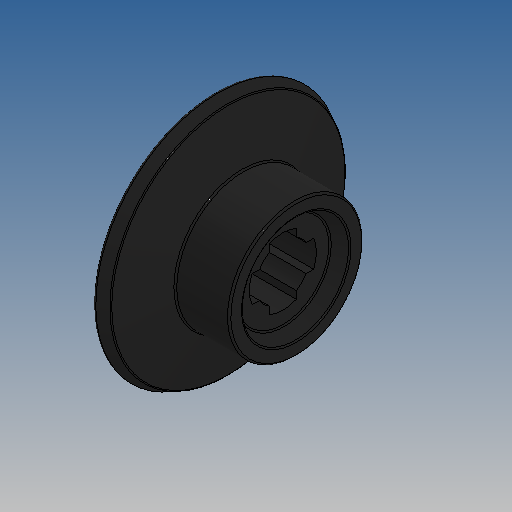
# Autodesk Inventor part: 50254-Black
Saved by Autodesk Inventor 2025 (Build 290162010, 162A)
## iProperties
Created: 2024-11-16
Part Number: 50254-Black
Material: ABS-Kunststoff
Document SubType Name: Modeling
Designer: hp.muther
Density: 1.06 g/cm^3
Appearance: Black
Author: hp.muther
Autodesk Inventor part; units mm, degrees
ref_plane "YZ Plane" through (0, 0, 0) normal (1, 0, 0) x (0, 1, 0)
ref_plane "XZ Plane" through (0, 0, 0) normal (0, 1, 0) x (-1, 0, 0)
ref_plane "XY Plane" through (0, 0, 0) normal (0, 0, 1) x (1, 0, 0)
sketch "Skizze1" plane through (0, 0, 0) normal (0, 1, 0) x (-1, 0, 0)
  line L0 (0, 0) -> (0, 7.2)
  line L1 (-0.1446, 7.2895) -> (-0.7422, 6.9916)
  line L2 (-0.7422, 6.9916) -> (-1.6, 4)
  line L3 (-1.6, 4) -> (-4.8, 4)
  line L4 (-4.8, 4) -> (-4.8, 0)
  line L5 (-4.8, 0) -> (0, 0)
  arc A0 (0, 7.2) -> (-0.1446, 7.2895) centre (-0.1, 7.2) ccw
  line L6 (-4.8, 3.1989) -> (-4, 2.8)
  line L7 (-4, 2.8) -> (-4, 0)
  line L8 (0, 2.4) -> (-0.7, 2.4)
  line L9 (-0.7979, 2.5201) -> (0, 6.4)
  arc A1 (-0.7979, 2.5201) -> (-0.7, 2.4) centre (-0.7, 2.5) ccw
  line L10 (0, 1.6) -> (-4, 1.6)
  dimension "d0" = 0.1
  dimension "d1" = 14.6
  dimension "d2" = 8
  dimension "d3" = 4.8
  dimension "d4" = 3.2
  dimension "d5" = 63.5
  dimension "d6" = 106
  dimension "d9" = 4.8
  dimension "d10" = 0.1
  dimension "d11" = 0.8
  dimension "d12" = 12.8
  dimension "d13" = 0.8
  dimension "d14" = 26.5
  dimension "d15" = 5.6
  dimension "d16" = 3.2
  constraints: 22 end point, 6 point on line, 4 point on circle, 4 tangent, 3 perpendicular, 2 centre point, 2 vertical, 1 horizontal, 1 parallel
  measures "d0" radius of A0
  measures "d2" diameter of L3 L5
  measures "d3" distance of L4.end L0.start
  measures "d4" distance of L2.end L3.end
  measures "d5" angle of L0 L1
  measures "d6" angle of L3 L2
  measures "d9" diameter of L8 L5
  measures "d10" radius of A1
  measures "d12" diameter of L9.end L5
  measures "d13" distance between parallel lines of L4 L7
  measures "d14" angle of L5 L6
  measures "d15" diameter of L6.end L5
  measures "d16" diameter of L10 L5
revolve "Umdrehung1" add sketch "Skizze1" angle 360 about axis through (4.8, 0, 0) along (-1, 0, 0) contours L10 L7 L6 L4 L3 L2 L1 A0 L0 L9 A1 L8
fillet "Rundung1" radius 0.1 7 edges at (4.8, 0, -4) (1.6, 0, -4) (0.7422, 0, -6.9916) (4.8, 0, -3.1989) (4, 0, -2.8) (0, 0, -2.4) (0, 0, -6.4)
sketch "Skizze2" plane through (0, 0, 0) normal (-1, 0, 0) x (0, 0, 1)
  circle A0 centre (0, 0) radius 2.3 projected
  line L0 (0, -0.8) -> (0, 0.8)
  line L1 (0, 0.8) -> (1.833, 0.8)
  arc A1 (1.833, -0.8) -> (1.833, 0.8) centre (0, 0) ccw
  line L2 (0, -0.8) -> (1.833, -0.8)
  circle A2 centre (0, 0) radius 1.6 projected
  dimension "d17" = 1.6
  dimension "d18" = 2
  constraints: 6 end point, 2 point on circle, 1 centre point, 1 coincident, 1 concentric, 1 horizontal, 1 midpoint, 1 perpendicular, 1 vertical
  measures "d17" distance between parallel lines of L1 L2
  measures "d18" radius of A1
extrude "Extrusion1" cut sketch "Skizze2" against normal blind 10 contours L0 L1 A2 L2 | A2 L1 A1 L2 picked at (0.5333, 0)
pattern_circular "Runde Anordnung1" count 4 over 360 about axis through (2, 0, 0) along (-1, 0, 0) of "Extrusion1"
equation "\"d13\" = d11"
